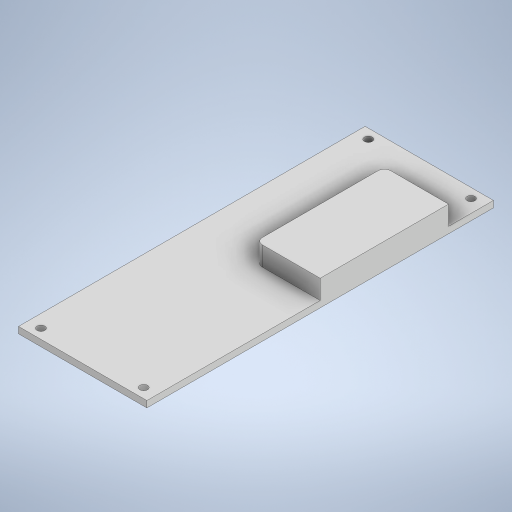
# Autodesk Inventor part: side_front
Saved by Autodesk Inventor 2024 (Build 280153000, 153)
## iProperties
Created: 2026-03-15
Part Number: side_front
Material: Generic
Document SubType Name: Modeling
Designer: HP
Density: 1 g/cm^3
Appearance: Default
Author: HP
Autodesk Inventor part; units mm, degrees
ref_plane "YZ Plane" through (0, 0, 0) normal (1, 0, 0) x (0, 1, 0)
ref_plane "XZ Plane" through (0, 0, 0) normal (0, 1, 0) x (-1, 0, 0)
ref_plane "XY Plane" through (0, 0, 0) normal (0, 0, 1) x (1, 0, 0)
sketch "Sketch1" plane through (0, 0, 0) normal (0, 1, 0) x (-1, 0, 0)
  line L0 (0, 0) -> (0, 135)
  line L1 (0, 135) -> (0, -135)
  line L2 (0, -135) -> (50, -135)
  line L3 (50, -135) -> (-50, -135)
  line L4 (-50, -135) -> (-50, 135)
  line L5 (-50, 135) -> (50, 135)
  line L6 (50, 135) -> (50, -135)
  line L7 (50, 135) -> (50, 127.5)
  line L8 (50, 127.5) -> (40, 127.5)
  circle A0 centre (40, 127.5) radius 3
  line L9 (40, 127.5) -> (-40, 127.5)
  circle A1 centre (-40, 127.5) radius 3
  line L10 (50, 0) -> (-50, 0)
  circle A2 centre (40, -127.5) radius 3
  circle A3 centre (-40, -127.5) radius 3
  dimension "d0" = 135
  dimension "d1" = 270
  dimension "d2" = 50
  dimension "d3" = 100
  dimension "d4" = 7.5
  dimension "d5" = 10
  dimension "d6" = 6
  dimension "d7" = 80
  dimension "d8" = 6
  constraints: 22 end point, 4 centre point, 4 perpendicular, 3 point on line, 2 coincident, 2 horizontal, 2 midpoint, 2 symmetric about line, 1 vertical, 2 other
  measures "d0" distance of L0.start L0.end
  measures "d1" distance of L0.end L1.end
  measures "d2" distance of L1.end L2.end
  measures "d3" distance of L2.end L3.end
  measures "d4" distance of L5.end L7.end
  measures "d5" distance of L7.end L8.end
  measures "d6" diameter of A0
  measures "d7" distance of L9.start L9.end
  measures "d8" diameter of A1
extrude "Extrusion1" add sketch "Sketch1" along normal blind 5 contours L10 L4 L5 L0 | L10 L6 L2 L1 | L0 L9 A0 L8 L6 L10 | L1 L3 L4 L10 | L0 L5 L6 L8 A0 L9
sketch "Sketch2" plane through (0, 5, 0) normal (0, 1, 0) x (1, 0, 0)
  line L0 (0, 0) -> (50, 0)
  line L1 (50, -135) -> (50, 135) projected
  line L2 (50, 0) -> (50, 100)
  line L3 (50, 100) -> (0, 100)
  line L4 (0, 100) -> (0, 0)
  dimension "d11" = 100
  constraints: 8 end point, 2 perpendicular, 1 midpoint, 1 vertical
  measures "d11" distance of L0.end L2.end
extrude "Extrusion2" add sketch "Sketch2" along normal blind 15
fillet "Fillet1" radius 5 1 edges at (0, 12.5, -100)
fillet "Fillet2" radius 5 1 edges at (0, 12.5, 0)
sketch "Sketch3" plane through (50, 5, -100) normal (0, 0, -1) x (-1, 0, 0)
  line L0 (0, 0) -> (0, 15) projected
  line L1 (0, 0) -> (0, 7.5)
  line L2 (0, 7.5) -> (20, 7.5)
  circle A0 centre (20, 7.5) radius 2.5
  point P0 (50, -5)
  dimension "d16" = 7.5
  dimension "d17" = 20
  dimension "d18" = 5
  constraints: 4 end point, 1 centre point, 1 coincident, 1 midpoint, 1 perpendicular
  measures "d16" distance of L0.start L1.end
  measures "d17" distance of L1.end L2.end
  measures "d18" diameter of A0
hole "Hole1" at (30, 12.5, -100) direction (0, 0, 1) diameter 6 depth 20 tip angle 118
sketch "Sketch4" plane through (0, 0, 0) normal (0, -1, 0) x (1, 0, 0)
  line L0 (50, -135) -> (-50, -135) projected
  line L1 (50, -135) -> (33, -135)
  line L2 (33, -135) -> (33, -100)
  line L3 (5, -100) -> (50, -100) projected
  line L4 (33, -100) -> (40, -100)
  line L5 (40, -100) -> (23, -100)
  line L6 (23, -100) -> (23, -50)
  line L7 (23, -50) -> (40, -50)
  line L8 (40, -50) -> (40, -100)
  line L9 (40, -100) -> (40, -95)
  line L10 (40, -95) -> (23, -95)
  line L11 (23, -95) -> (23, -100)
  point P0 (0, 0)
  dimension "d26" = 17
  dimension "d27" = 35
  dimension "d28" = 7
  dimension "d29" = 17
  dimension "d30" = 50
  dimension "d31" = 5
  constraints: 20 end point, 6 point on line, 4 perpendicular, 1 collinear
  measures "d26" distance of L0.start L1.end
  measures "d27" distance of L1.end L2.end
  measures "d28" distance of L2.end L4.end
  measures "d29" distance of L4.end L5.end
  measures "d30" distance of L5.end L6.end
  measures "d31" distance of L4.end L9.end
extrude "Extrusion3" cut sketch "Sketch4" against normal blind 16 contours L6 L7 L8 L10
body "Solid1"
